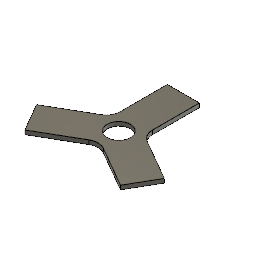
Propstop8mm (Autodesk Fusion 360 design; units mm, degrees)
Autodesk Fusion 360 part; units mm, degrees
sketch "Skizze1" plane through (0, 0, 0) normal (0, 1, 0) x (1, 0, 0)
  line L0 (-5.75, 0) -> (5.75, 0)
  line L1 (5.75, 0) -> (5.75, 23)
  line L2 (5.75, 23) -> (-5.75, 23)
  line L3 (-5.75, 23) -> (-5.75, 0)
  circle A0 centre (0, 0) radius 4.1
  line L4 (-2.875, 4.9796) -> (-22.7936, -6.5204)
  line L5 (2.875, -4.9796) -> (-2.875, 4.9796)
  circle A1 centre (0, 0) radius 4.1
  line L6 (-22.7936, -6.5204) -> (-17.0436, -16.4796)
  line L7 (-17.0436, -16.4796) -> (2.875, -4.9796)
  line L8 (-2.875, -4.9796) -> (17.0436, -16.4796)
  line L9 (2.875, 4.9796) -> (-2.875, -4.9796)
  circle A2 centre (0, 0) radius 4.1
  line L10 (17.0436, -16.4796) -> (22.7936, -6.5204)
  line L11 (22.7936, -6.5204) -> (2.875, 4.9796)
  dimension "d1" = 8.2
  dimension "d2" = 11.5
  dimension "d3" = 23
  dimension "d4" = 5.75
  dimension "d8" = 360
  constraint horizontal L0
  constraint vertical L1
  constraint horizontal L2
  constraint vertical L3
  constraint coincident A0.centre A1.centre
  constraint coincident A0.centre L0
  measures "d1" diameter of A0
  measures "d2" distance of L1.end L2.end
  measures "d3" distance of L0.end L1.end
  measures "d4" distance of A0.centre L1
extrude "Extrusion1" add sketch "Skizze1" along normal blind 1.5 contours L0 L1 A0 A1 L9 A2 L11 | L0 L1 A0 L5 A1 L7 L8 A2 L10 L11 | L1 L2 L3 A0 L4 L5 A1 L9 A2 L11 | A0 L5 A1 L7 L8 L9 A2 | L0 L3 A0 L4 A1 L6 L7 L8 L9 A2 | L0 L3 A0 L4 L5 A1 A2
fillet "Abrundung1" radius 5 3 edges at (0, 0.75, 6.6395) (5.75, 0.75, -3.3198) (-5.75, 0.75, -3.3198)
equation "d4 = d2 / 2"
